Autodesk Fusion 360 part; units mm, degrees
(part 5 of 8)
  spline S1362 degree 3 poles (9.3996, -113.8343) (9.4042, -113.7081) (9.4002, -113.5528) (9.3979, -113.4927) knots 0 0 0 0 1 1 1 1
  spline S1363 degree 3 poles (9.3979, -113.4927) (9.3922, -113.4256) (9.399, -113.3996) (9.4154, -113.4303) knots 0 0 0 0 1 1 1 1
  spline S1364 degree 3 poles (9.4154, -113.4303) (9.4289, -113.4588) (9.4314, -113.4384) (9.4148, -113.3851) knots 0 0 0 0 1 1 1 1
  spline S1365 degree 3 poles (9.4148, -113.3851) (9.401, -113.334) (9.4015, -113.2762) (9.4145, -113.2595) knots 0 0 0 0 1 1 1 1
  spline S1366 degree 3 poles (9.4145, -113.2595) (9.4297, -113.24) (9.4323, -113.1794) (9.4222, -113.1178) knots 0 0 0 0 1 1 1 1
  spline S1367 degree 3 poles (9.4222, -113.1178) (9.4128, -113.0611) (9.4025, -112.9367) (9.4036, -112.8436) knots 0 0 0 0 1 1 1 1
  spline S1368 degree 3 poles (9.4036, -112.8436) (9.4042, -112.7455) (9.4014, -112.6001) (9.396, -112.5153) knots 0 0 0 0 1 1 1 1
  spline S1369 degree 3 poles (9.396, -112.5153) (9.3934, -112.4327) (9.3982, -112.3693) (9.4065, -112.3758) knots 0 0 0 0 1 1 1 1
  spline S1370 degree 3 poles (9.4065, -112.3758) (9.4176, -112.3845) (9.4227, -112.3437) (9.4154, -112.2842) knots 0 0 0 0 1 1 1 1
  spline S1371 degree 3 poles (9.4154, -112.2842) (9.4045, -112.1549) (9.4262, -112.1271) (9.5265, -112.1248) knots 0 0 0 0 1 1 1 1
  spline S1372 degree 3 poles (9.5265, -112.1248) (9.5992, -112.1234) (9.5964, -112.1213) (9.507, -112.1096) knots 0 0 0 0 1 1 1 1
  spline S1373 degree 3 poles (9.507, -112.1096) (9.4149, -112.0958) (9.4065, -112.0893) (9.3994, -111.9494) knots 0 0 0 0 1 1 1 1
  spline S1374 degree 3 poles (9.3994, -111.9494) (9.3946, -111.8696) (9.3998, -111.7885) (9.4106, -111.7746) knots 0 0 0 0 1 1 1 1
  spline S1375 degree 3 poles (9.4106, -111.7746) (9.4236, -111.7579) (9.4203, -111.7106) (9.405, -111.6672) knots 0 0 0 0 1 1 1 1
  spline S1376 degree 3 poles (9.405, -111.6672) (9.3896, -111.6239) (9.3885, -111.5738) (9.4037, -111.5543) knots 0 0 0 0 1 1 1 1
  spline S1377 degree 3 poles (9.4037, -111.5543) (9.4189, -111.5349) (9.4199, -111.4819) (9.4067, -111.4358) knots 0 0 0 0 1 1 1 1
  spline S1378 degree 3 poles (9.4067, -111.4358) (9.3935, -111.3897) (9.3902, -111.3423) (9.4011, -111.3284) knots 0 0 0 0 1 1 1 1
  spline S1379 degree 3 poles (9.4011, -111.3284) (9.4184, -111.3062) (9.4189, -111.2483) (9.4093, -111.0887) knots 0 0 0 0 1 1 1 1
  spline S1380 degree 3 poles (9.4093, -111.0887) (9.3971, -110.8866) (9.398, -110.5874) (9.4111, -110.5707) knots 0 0 0 0 1 1 1 1
  spline S1381 degree 3 poles (9.4111, -110.5707) (9.4176, -110.5624) (9.4208, -110.5067) (9.4185, -110.4467) knots 0 0 0 0 1 1 1 1
  spline S1382 degree 3 poles (9.4185, -110.4467) (9.406, -110.325) (9.4061, -110.2848) (9.3975, -109.9692) knots 0 0 0 0 1 1 1 1
  spline S1383 degree 3 poles (9.3975, -109.9692) (9.3922, -109.8442) (9.3981, -109.7279) (9.4068, -109.7167) knots 0 0 0 0 1 1 1 1
  spline S1384 degree 3 poles (9.4068, -109.7167) (9.4154, -109.7056) (9.4159, -109.6478) (9.4036, -109.589) knots 0 0 0 0 1 1 1 1
  spline S1385 degree 3 poles (9.4036, -109.589) (9.3942, -109.5323) (9.3967, -109.5119) (9.4102, -109.5404) knots 0 0 0 0 1 1 1 1
  spline S1386 degree 3 poles (9.4102, -109.5404) (9.426, -109.5661) (9.4282, -109.5231) (9.4207, -109.4411) knots 0 0 0 0 1 1 1 1
  spline S1387 degree 3 poles (9.4207, -109.4411) (9.3888, -109.161) (9.385, -109.1715) (9.5373, -109.1428) knots 0 0 0 0 1 1 1 1
  spline S1388 degree 3 poles (9.5373, -109.1428) (9.611, -109.1287) (9.6373, -109.1179) (9.5971, -109.1178) knots 0 0 0 0 1 1 1 1
  spline S1389 degree 3 poles (9.5971, -109.1178) (9.5569, -109.1178) (9.5136, -109.0929) (9.5056, -109.0688) knots 0 0 0 0 1 1 1 1
  spline S1390 degree 3 poles (9.5056, -109.0688) (9.4949, -109.0424) (9.4871, -109.0409) (9.483, -109.069) knots 0 0 0 0 1 1 1 1
  spline S1391 degree 3 poles (9.483, -109.069) (9.473, -109.1507) (9.4047, -109.1063) (9.3981, -109.0116) knots 0 0 0 0 1 1 1 1
  spline S1392 degree 3 poles (9.3981, -109.0116) (9.3942, -108.9593) (9.3998, -108.9234) (9.4109, -108.9321) knots 0 0 0 0 1 1 1 1
  spline S1393 degree 3 poles (9.4109, -108.9321) (9.4221, -108.9408) (9.4209, -108.8907) (9.4096, -108.8192) knots 0 0 0 0 1 1 1 1
  spline S1394 degree 3 poles (9.4096, -108.8192) (9.3983, -108.7477) (9.4, -108.6997) (9.4139, -108.7106) knots 0 0 0 0 1 1 1 1
  spline S1395 degree 3 poles (9.4139, -108.7106) (9.4278, -108.7214) (9.4235, -108.6868) (9.4097, -108.6357) knots 0 0 0 0 1 1 1 1
  spline S1396 degree 3 poles (9.4097, -108.6357) (9.3937, -108.5874) (9.392, -108.5323) (9.405, -108.5156) knots 0 0 0 0 1 1 1 1
  spline S1397 degree 3 poles (9.405, -108.5156) (9.4181, -108.4989) (9.4219, -108.4482) (9.4136, -108.4015) knots 0 0 0 0 1 1 1 1
  spline S1398 degree 3 poles (9.4136, -108.4015) (9.4054, -108.3547) (9.4002, -108.1895) (9.4033, -108.0308) knots 0 0 0 0 1 1 1 1
  spline S1399 degree 3 poles (9.4033, -108.0308) (9.4037, -107.8699) (9.3981, -107.7223) (9.3929, -107.7003) knots 0 0 0 0 1 1 1 1
  spline S1400 degree 3 poles (9.3929, -107.7003) (9.3843, -107.6712) (9.3908, -107.6629) (9.4103, -107.6781) knots 0 0 0 0 1 1 1 1
  spline S1401 degree 3 poles (9.4103, -107.6781) (9.4242, -107.6889) (9.4316, -107.6679) (9.4218, -107.6289) knots 0 0 0 0 1 1 1 1
  spline S1402 degree 3 poles (9.4218, -107.6289) (9.3982, -107.5388) (9.3926, -106.8584) (9.4148, -106.8758) knots 0 0 0 0 1 1 1 1
  spline S1403 degree 3 poles (9.4148, -106.8758) (9.4259, -106.8845) (9.4205, -106.8399) (9.4048, -106.774) knots 0 0 0 0 1 1 1 1
  spline S1404 degree 3 poles (9.4048, -106.774) (9.3898, -106.713) (9.3924, -106.6523) (9.4116, -106.645) knots 0 0 0 0 1 1 1 1
  spline S1405 degree 3 poles (9.4116, -106.645) (9.4336, -106.6397) (9.4339, -106.6221) (9.4145, -106.6069) knots 0 0 0 0 1 1 1 1
  spline S1406 degree 3 poles (9.4145, -106.6069) (9.3894, -106.5874) (9.396, -106.579) (9.4449, -106.568) knots 0 0 0 0 1 1 1 1
  spline S1407 degree 3 poles (9.4449, -106.568) (9.4987, -106.5564) (9.4953, -106.5492) (9.4338, -106.5191) knots 0 0 0 0 1 1 1 1
  spline S1408 degree 3 poles (9.4338, -106.5191) (9.3912, -106.4992) (9.3717, -106.484) (9.3888, -106.4794) knots 0 0 0 0 1 1 1 1
  spline S1409 degree 3 poles (9.3888, -106.4794) (9.4036, -106.4776) (9.4125, -106.386) (9.4013, -106.2743) knots 0 0 0 0 1 1 1 1
  spline S1410 degree 3 poles (9.4013, -106.2743) (9.3928, -106.1647) (9.3977, -106.0611) (9.4151, -106.0388) knots 0 0 0 0 1 1 1 1
  spline S1411 degree 3 poles (9.4151, -106.0388) (9.4303, -106.0194) (9.4322, -105.994) (9.4183, -105.9832) knots 0 0 0 0 1 1 1 1
  spline S1412 degree 3 poles (9.4183, -105.9832) (9.3877, -105.9593) (9.3954, -105.2848) (9.4254, -105.2635) knots 0 0 0 0 1 1 1 1
  spline S1413 degree 3 poles (9.4254, -105.2635) (9.4397, -105.2567) (9.44, -105.2391) (9.4261, -105.2282) knots 0 0 0 0 1 1 1 1
  spline S1414 degree 3 poles (9.4261, -105.2282) (9.3733, -105.187) (9.3985, -104.6963) (9.4496, -104.6825) knots 0 0 0 0 1 1 1 1
  spline S1415 degree 3 poles (9.4496, -104.6825) (9.4815, -104.676) (9.5088, -104.6526) (9.5212, -104.631) knots 0 0 0 0 1 1 1 1
  spline S1416 degree 3 poles (11.4691, -103.9771) (11.4765, -103.9963) (11.5151, -104.0041) (11.5542, -103.9943) knots 0 0 0 0 1 1 1 1
  spline S1417 degree 3 poles (11.5542, -103.9943) (11.6179, -103.9814) (11.6223, -103.9759) (11.5687, -103.9699) knots 0 0 0 0 1 1 1 1
  spline S1418 degree 3 poles (11.5687, -103.9699) (11.5152, -103.9639) (11.5174, -103.9611) (11.5833, -103.9455) knots 0 0 0 0 1 1 1 1
  spline S1419 degree 3 poles (11.5833, -103.9455) (11.6713, -103.9246) (11.7334, -103.9597) (11.6637, -103.9859) knots 0 0 0 0 1 1 1 1
  spline S1420 degree 3 poles (11.6637, -103.9859) (11.6281, -104.0028) (11.6336, -104.0072) (11.6832, -104.0011) knots 0 0 0 0 1 1 1 1
  spline S1421 degree 3 poles (11.6832, -104.0011) (11.7206, -103.999) (11.7612, -103.9814) (11.7742, -103.9648) knots 0 0 0 0 1 1 1 1
  spline S1422 degree 3 poles (11.7742, -103.9648) (11.7872, -103.9481) (11.8191, -103.9417) (11.8479, -103.9507) knots 0 0 0 0 1 1 1 1
  spline S1423 degree 3 poles (11.8479, -103.9507) (11.8794, -103.9619) (11.8785, -103.9746) (11.8422, -103.9866) knots 0 0 0 0 1 1 1 1
  spline S1424 degree 3 poles (11.8422, -103.9866) (11.7995, -104.0069) (11.8023, -104.0091) (11.8672, -104.0061) knots 0 0 0 0 1 1 1 1
  spline S1425 degree 3 poles (11.8672, -104.0061) (11.9124, -104.0056) (11.9437, -103.9942) (11.9419, -103.9794) knots 0 0 0 0 1 1 1 1
  spline S1426 degree 3 poles (11.9419, -103.9794) (11.9404, -103.9469) (12.0531, -103.923) (12.0864, -103.9491) knots 0 0 0 0 1 1 1 1
  spline S1427 degree 3 poles (12.0864, -103.9491) (12.1003, -103.9599) (12.0944, -103.9732) (12.0731, -103.9834) knots 0 0 0 0 1 1 1 1
  spline S1428 degree 3 poles (12.0731, -103.9834) (12.0105, -104.0061) (12.0519, -104.0161) (12.1327, -103.9987) knots 0 0 0 0 1 1 1 1
  spline S1429 degree 3 poles (12.1327, -103.9987) (12.1987, -103.983) (12.2008, -103.9802) (12.1473, -103.9742) knots 0 0 0 0 1 1 1 1
  spline S1430 degree 3 poles (12.1473, -103.9742) (12.0938, -103.9683) (12.096, -103.9655) (12.1619, -103.9498) knots 0 0 0 0 1 1 1 1
  spline S1431 degree 3 poles (12.1619, -103.9498) (12.2399, -103.9302) (12.3141, -103.9613) (12.2494, -103.9868) knots 0 0 0 0 1 1 1 1
  spline S1432 degree 3 poles (12.2494, -103.9868) (12.1797, -104.013) (12.2283, -104.0196) (12.3338, -103.9991) knots 0 0 0 0 1 1 1 1
  spline S1433 degree 3 poles (12.3338, -103.9991) (12.4344, -103.9792) (12.4366, -103.9764) (12.3484, -103.9747) knots 0 0 0 0 1 1 1 1
  spline S1434 degree 3 poles (12.3484, -103.9747) (12.2603, -103.9729) (12.2624, -103.9702) (12.363, -103.9503) knots 0 0 0 0 1 1 1 1
  spline S1435 degree 3 poles (12.363, -103.9503) (12.4686, -103.9298) (12.5471, -103.9553) (12.4682, -103.9876) knots 0 0 0 0 1 1 1 1
  spline S1436 degree 3 poles (12.4682, -103.9876) (12.4319, -103.9996) (12.4403, -104.0061) (12.4932, -104.0072) knots 0 0 0 0 1 1 1 1
  spline S1437 degree 3 poles (12.4932, -104.0072) (12.5356, -104.0045) (12.5761, -103.9869) (12.5842, -103.9709) knots 0 0 0 0 1 1 1 1
  spline S1438 degree 3 poles (12.5842, -103.9709) (12.5945, -103.952) (12.6236, -103.9434) (12.6523, -103.9525) knots 0 0 0 0 1 1 1 1
  spline S1439 degree 3 poles (12.6523, -103.9525) (12.6839, -103.9637) (12.6829, -103.9763) (12.6495, -103.9905) knots 0 0 0 0 1 1 1 1
  spline S1440 degree 3 poles (12.6495, -103.9905) (12.6182, -104.0019) (12.6392, -104.0094) (12.6965, -104.0048) knots 0 0 0 0 1 1 1 1
  spline S1441 degree 3 poles (12.6965, -104.0048) (12.7515, -104.0031) (12.802, -103.9843) (12.8144, -103.9627) knots 0 0 0 0 1 1 1 1
  spline S1442 degree 3 poles (12.8144, -103.9627) (12.8247, -103.9439) (12.8528, -103.9479) (12.8779, -103.9675) knots 0 0 0 0 1 1 1 1
  spline S1443 degree 3 poles (12.8779, -103.9675) (12.9035, -103.992) (12.9267, -103.9967) (12.927, -103.979) knots 0 0 0 0 1 1 1 1
  spline S1444 degree 3 poles (12.927, -103.979) (12.9336, -103.9305) (13.0725, -103.936) (13.0737, -103.9862) knots 0 0 0 0 1 1 1 1
  spline S1445 degree 3 poles (13.0737, -103.9862) (13.0871, -104.3414) (13.0769, -104.5035) (13.0385, -104.5183) knots 0 0 0 0 1 1 1 1
  spline S1446 degree 3 poles (13.0385, -104.5183) (13.0121, -104.529) (13.0106, -104.5368) (13.0338, -104.5415) knots 0 0 0 0 1 1 1 1
  spline S1447 degree 3 poles (13.0338, -104.5415) (13.0669, -104.5449) (13.0985, -106.3783) (13.0691, -106.5075) knots 0 0 0 0 1 1 1 1
  spline S1448 degree 3 poles (13.0691, -106.5075) (13.0654, -106.518) (12.8203, -106.528) (12.526, -106.5264) knots 0 0 0 0 1 1 1 1
  spline S1449 degree 3 poles (12.526, -106.5264) (12.2318, -106.5249) (11.9861, -106.5299) (11.9818, -106.5355) knots 0 0 0 0 1 1 1 1
  spline S1450 degree 3 poles (11.9818, -106.5355) (11.9753, -106.5438) (12.0365, -106.5514) (12.117, -106.5515) knots 0 0 0 0 1 1 1 1
  spline S1451 degree 3 poles (12.117, -106.5515) (12.2023, -106.5511) (12.2735, -106.5575) (12.2846, -106.5661) knots 0 0 0 0 1 1 1 1
  spline S1452 degree 3 poles (12.2846, -106.5661) (12.293, -106.5727) (12.3018, -106.9109) (12.3059, -107.3125) knots 0 0 0 0 1 1 1 1
  spline S1453 degree 3 poles (12.3059, -107.3125) (12.3107, -107.7819) (12.333, -108.0857) (12.3678, -108.1443) knots 0 0 0 0 1 1 1 1
  spline S1454 degree 3 poles (12.3678, -108.1443) (12.3965, -108.1936) (12.5461, -108.4089) (12.7028, -108.6209) knots 0 0 0 0 1 1 1 1
  spline S1455 degree 3 poles (12.7028, -108.6209) (12.8546, -108.8335) (12.9902, -109.038) (12.9951, -109.0776) knots 0 0 0 0 1 1 1 1
  spline S1456 degree 3 poles (12.9951, -109.0776) (13.007, -109.1541) (12.959, -109.1926) (12.546, -109.4519) knots 0 0 0 0 1 1 1 1
  spline S1457 degree 3 poles (12.546, -109.4519) (12.3895, -109.5491) (12.3055, -109.6222) (12.2961, -109.6686) knots 0 0 0 0 1 1 1 1
  spline S1458 degree 3 poles (12.2961, -109.6686) (12.2855, -109.7051) (12.3057, -109.9715) (12.3403, -110.2538) knots 0 0 0 0 1 1 1 1
  line L112 (12.3403, -110.2538) -> (12.3986, -110.7694)
  line L113 (12.3986, -110.7694) -> (12.6643, -111.2143)
  line L114 (12.6643, -111.2143) -> (12.9273, -111.657)
  line L115 (12.9273, -111.657) -> (12.9828, -112.1704)
  spline S1459 degree 3 poles (12.9828, -112.1704) (13.0278, -112.5369) (13.028, -112.7027) (12.9911, -112.75) knots 0 0 0 0 1 1 1 1
  spline S1460 degree 3 poles (12.9911, -112.75) (12.9607, -112.7889) (12.7218, -112.9514) (12.4554, -113.1148) knots 0 0 0 0 1 1 1 1
  spline S1461 degree 3 poles (12.4554, -113.1148) (12.126, -113.3186) (11.9599, -113.4395) (11.9205, -113.5072) knots 0 0 0 0 1 1 1 1
  spline S1462 degree 3 poles (11.9205, -113.5072) (11.8605, -113.6126) (11.7411, -114.2983) (11.7541, -114.4651) knots 0 0 0 0 1 1 1 1
  spline S1463 degree 3 poles (11.7541, -114.4651) (11.7564, -114.5251) (11.7792, -114.5877) (11.8014, -114.605) knots 0 0 0 0 1 1 1 1
  spline S1464 degree 3 poles (11.8014, -114.605) (11.8264, -114.6246) (11.8217, -114.6478) (11.7889, -114.6669) knots 0 0 0 0 1 1 1 1
  spline S1465 degree 3 poles (11.7889, -114.6669) (11.7468, -114.6922) (11.7502, -114.6993) (11.7926, -114.6966) knots 0 0 0 0 1 1 1 1
  spline S1466 degree 3 poles (11.7926, -114.6966) (11.8752, -114.694) (12.6789, -116.1636) (12.6604, -116.279) knots 0 0 0 0 1 1 1 1
  spline S1467 degree 3 poles (12.6604, -116.279) (12.6538, -116.3275) (12.4805, -116.6353) (12.2799, -116.9666) knots 0 0 0 0 1 1 1 1
  spline S1468 degree 3 poles (12.2799, -116.9666) (12.0641, -117.3173) (11.9087, -117.6078) (11.9049, -117.6585) knots 0 0 0 0 1 1 1 1
  spline S1469 degree 3 poles (11.9049, -117.6585) (11.8973, -117.7197) (12.0151, -117.9415) (12.2824, -118.3787) knots 0 0 0 0 1 1 1 1
  spline S1470 degree 3 poles (12.2824, -118.3787) (12.735, -119.1173) (12.7463, -119.0053) (12.1724, -119.4478) knots 0 0 0 0 1 1 1 1
  spline S1471 degree 3 poles (12.1724, -119.4478) (11.789, -119.7437) (11.7111, -119.8261) (11.6907, -119.9668) knots 0 0 0 0 1 1 1 1
  spline S1472 degree 3 poles (11.6907, -119.9668) (11.6626, -120.106) (11.7858, -120.7619) (11.8564, -120.8663) knots 0 0 0 0 1 1 1 1
  spline S1473 degree 3 poles (11.8564, -120.8663) (11.9742, -121.0479) (12.5647, -122.1315) (12.5714, -122.186) knots 0 0 0 0 1 1 1 1
  spline S1474 degree 3 poles (12.5714, -122.186) (12.5756, -122.2206) (12.4475, -122.3846) (12.1544, -122.7197) knots 0 0 0 0 1 1 1 1
  spline S1475 degree 3 poles (12.1544, -122.7197) (11.8237, -123.0971) (11.7086, -123.2444) (11.643, -123.3857) knots 0 0 0 0 1 1 1 1
  spline S1476 degree 3 poles (11.643, -123.3857) (11.5694, -123.543) (11.4368, -123.7528) (11.4341, -123.7104) knots 0 0 0 0 1 1 1 1
  spline S1477 degree 3 poles (11.4341, -123.7104) (11.4295, -122.5473) (11.4436, -122.1912) (11.4873, -122.1582) knots 0 0 0 0 1 1 1 1
  spline S1478 degree 3 poles (11.4873, -122.1582) (11.5245, -122.1336) (11.5239, -122.1286) (11.4898, -122.1378) knots 0 0 0 0 1 1 1 1
  spline S1479 degree 3 poles (11.4898, -122.1378) (11.4536, -122.1498) (11.4365, -121.7649) (11.4348, -120.8502) knots 0 0 0 0 1 1 1 1
  spline S1480 degree 3 poles (11.4348, -120.8502) (11.4348, -119.8475) (11.4478, -119.5443) (11.4936, -119.5487) knots 0 0 0 0 1 1 1 1
  spline S1481 degree 3 poles (11.4936, -119.5487) (11.5388, -119.5482) (11.5382, -119.5432) (11.4912, -119.5289) knots 0 0 0 0 1 1 1 1
  spline S1482 degree 3 poles (11.4912, -119.5289) (11.4513, -119.5112) (11.4341, -119.453) (11.4328, -119.34) knots 0 0 0 0 1 1 1 1
  spline S1483 degree 3 poles (11.4328, -119.34) (11.4345, -119.2518) (11.4338, -118.7543) (11.4312, -118.2419) knots 0 0 0 0 1 1 1 1
  spline S1484 degree 3 poles (11.4312, -118.2419) (11.4303, -117.4981) (11.4447, -117.3079) (11.4926, -117.3095) knots 0 0 0 0 1 1 1 1
  spline S1485 degree 3 poles (11.4926, -117.3095) (11.5406, -117.3112) (11.5427, -117.3084) (11.4951, -117.2891) knots 0 0 0 0 1 1 1 1
  spline S1486 degree 3 poles (11.4951, -117.2891) (11.4509, -117.2769) (11.4364, -116.9746) (11.4365, -116.0749) knots 0 0 0 0 1 1 1 1
  spline S1487 degree 3 poles (11.4365, -116.0749) (11.4361, -115.4164) (11.4358, -114.0015) (11.435, -112.931) knots 0 0 0 0 1 1 1 1
  spline S1488 degree 3 poles (11.435, -112.931) (11.4349, -111.8654) (11.4321, -110.5739) (11.4351, -110.0659) knots 0 0 0 0 1 1 1 1
  spline S1489 degree 3 poles (11.4351, -110.0659) (11.4299, -109.3276) (11.4448, -109.1423) (11.4937, -109.1313) knots 0 0 0 0 1 1 1 1
  spline S1490 degree 3 poles (11.4937, -109.1313) (11.5448, -109.1174) (11.5464, -109.1097) (11.4994, -109.0954) knots 0 0 0 0 1 1 1 1
  spline S1491 degree 3 poles (11.4994, -109.0954) (11.4552, -109.0832) (11.438, -109.025) (11.4367, -108.9121) knots 0 0 0 0 1 1 1 1
  spline S1492 degree 3 poles (11.4367, -108.9121) (11.4356, -108.8217) (11.4349, -108.1809) (11.4358, -107.4922) knots 0 0 0 0 1 1 1 1
  spline S1493 degree 3 poles (11.4358, -107.4922) (11.4339, -106.8013) (11.4353, -105.728) (11.4342, -105.1048) knots 0 0 0 0 1 1 1 1
  spline S1494 degree 3 poles (11.4342, -105.1048) (11.4352, -104.4789) (11.4397, -103.9631) (11.4441, -103.9576) knots 0 0 0 0 1 1 1 1
  spline S1495 degree 3 poles (11.4441, -103.9576) (11.4506, -103.9492) (11.4617, -103.9579) (11.4691, -103.9771) knots 0 0 0 0 1 1 1 1
  spline S1496 degree 3 poles (10.2121, -106.2049) (10.2283, -106.2758) (10.2333, -106.2752) (10.2319, -106.2024) knots 0 0 0 0 1 1 1 1
  spline S1497 degree 3 poles (10.2319, -106.2024) (10.232, -106.1622) (10.2271, -106.1226) (10.2215, -106.1183) knots 0 0 0 0 1 1 1 1
  spline S1498 degree 3 poles (10.2215, -106.1183) (10.1993, -106.1009) (10.1958, -106.134) (10.2121, -106.2049) knots 0 0 0 0 1 1 1 1
  spline S1499 degree 3 poles (9.9148, -109.1467) (9.9204, -109.151) (9.96, -109.1462) (10.0012, -109.1336) knots 0 0 0 0 1 1 1 1
  spline S1500 degree 3 poles (10.0012, -109.1336) (10.0699, -109.1201) (10.0693, -109.1152) (9.9966, -109.1165) knots 0 0 0 0 1 1 1 1
  spline S1501 degree 3 poles (9.9966, -109.1165) (9.9238, -109.1179) (9.8926, -109.1293) (9.9148, -109.1467) knots 0 0 0 0 1 1 1 1
  spline S1502 degree 3 poles (9.4857, -110.1142) (9.502, -110.1851) (9.5069, -110.1845) (9.5055, -110.1118) knots 0 0 0 0 1 1 1 1
  spline S1503 degree 3 poles (9.5055, -110.1118) (9.5056, -110.0715) (9.5007, -110.0319) (9.4952, -110.0276) knots 0 0 0 0 1 1 1 1
  spline S1504 degree 3 poles (9.4952, -110.0276) (9.4729, -110.0102) (9.4695, -110.0433) (9.4857, -110.1142) knots 0 0 0 0 1 1 1 1
  spline S1505 degree 3 poles (10.2155, -110.3262) (10.2317, -110.3971) (10.2366, -110.3965) (10.2353, -110.3238) knots 0 0 0 0 1 1 1 1
  spline S1506 degree 3 poles (10.2353, -110.3238) (10.2353, -110.2835) (10.2305, -110.2439) (10.2249, -110.2396) knots 0 0 0 0 1 1 1 1
  spline S1507 degree 3 poles (10.2249, -110.2396) (10.2027, -110.2222) (10.1992, -110.2553) (10.2155, -110.3262) knots 0 0 0 0 1 1 1 1
  spline S1508 degree 3 poles (9.7288, -112.1352) (9.7344, -112.1395) (9.774, -112.1346) (9.8152, -112.122) knots 0 0 0 0 1 1 1 1
  spline S1509 degree 3 poles (9.8152, -112.122) (9.8839, -112.1086) (9.8833, -112.1036) (9.8106, -112.105) knots 0 0 0 0 1 1 1 1
  spline S1510 degree 3 poles (9.8106, -112.105) (9.7379, -112.1064) (9.7066, -112.1178) (9.7288, -112.1352) knots 0 0 0 0 1 1 1 1
  spline S1511 degree 3 poles (9.4874, -113.6074) (9.5036, -113.6783) (9.5086, -113.6777) (9.5072, -113.605) knots 0 0 0 0 1 1 1 1
  spline S1512 degree 3 poles (9.5072, -113.605) (9.5058, -113.5323) (9.4944, -113.501) (9.477, -113.5232) knots 0 0 0 0 1 1 1 1
  spline S1513 degree 3 poles (9.477, -113.5232) (9.4727, -113.5288) (9.4776, -113.5684) (9.4874, -113.6074) knots 0 0 0 0 1 1 1 1
  spline S1514 degree 3 poles (9.4865, -114.0096) (9.5027, -114.0805) (9.5077, -114.0799) (9.5063, -114.0072) knots 0 0 0 0 1 1 1 1
  spline S1515 degree 3 poles (9.5063, -114.0072) (9.5064, -113.967) (9.5015, -113.9274) (9.496, -113.923) knots 0 0 0 0 1 1 1 1
  spline S1516 degree 3 poles (9.496, -113.923) (9.4737, -113.9057) (9.4703, -113.9387) (9.4865, -114.0096) knots 0 0 0 0 1 1 1 1
  spline S1517 degree 3 poles (9.4856, -114.4119) (9.5019, -114.4828) (9.5068, -114.4821) (9.5054, -114.4094) knots 0 0 0 0 1 1 1 1
  spline S1518 degree 3 poles (9.5054, -114.4094) (9.504, -114.3367) (9.4927, -114.3054) (9.4753, -114.3277) knots 0 0 0 0 1 1 1 1
  spline S1519 degree 3 poles (9.4753, -114.3277) (9.4709, -114.3332) (9.4758, -114.3729) (9.4856, -114.4119) knots 0 0 0 0 1 1 1 1
  spline S1520 degree 3 poles (9.9086, -114.8274) (9.9142, -114.8317) (9.9538, -114.8269) (9.995, -114.8143) knots 0 0 0 0 1 1 1 1
  spline S1521 degree 3 poles (9.995, -114.8143) (10.0637, -114.8008) (10.0631, -114.7959) (9.9903, -114.7973) knots 0 0 0 0 1 1 1 1
  spline S1522 degree 3 poles (9.9903, -114.7973) (9.9176, -114.7986) (9.8864, -114.81) (9.9086, -114.8274) knots 0 0 0 0 1 1 1 1
  spline S1523 degree 3 poles (9.4882, -116.0703) (9.5044, -116.1412) (9.5094, -116.1406) (9.508, -116.0679) knots 0 0 0 0 1 1 1 1
  spline S1524 degree 3 poles (9.508, -116.0679) (9.5066, -115.9952) (9.4952, -115.9639) (9.4779, -115.9861) knots 0 0 0 0 1 1 1 1
  spline S1525 degree 3 poles (9.4779, -115.9861) (9.4735, -115.9917) (9.4784, -116.0313) (9.4882, -116.0703) knots 0 0 0 0 1 1 1 1
  spline S1526 degree 3 poles (9.489, -117.1006) (9.5053, -117.1715) (9.5102, -117.1709) (9.5088, -117.0982) knots 0 0 0 0 1 1 1 1
  spline S1527 degree 3 poles (9.5088, -117.0982) (9.5089, -117.058) (9.5041, -117.0184) (9.4985, -117.014) knots 0 0 0 0 1 1 1 1
  spline S1528 degree 3 poles (9.4985, -117.014) (9.4763, -116.9966) (9.4728, -117.0297) (9.489, -117.1006) knots 0 0 0 0 1 1 1 1
  spline S1529 degree 3 poles (10.2118, -116.2328) (10.2281, -116.3037) (10.233, -116.303) (10.2317, -116.2303) knots 0 0 0 0 1 1 1 1
  spline S1530 degree 3 poles (10.2317, -116.2303) (10.2303, -116.1576) (10.2189, -116.1263) (10.2015, -116.1486) knots 0 0 0 0 1 1 1 1
  spline S1531 degree 3 poles (10.2015, -116.1486) (10.1972, -116.1541) (10.202, -116.1938) (10.2118, -116.2328) knots 0 0 0 0 1 1 1 1
  spline S1532 degree 3 poles (9.4847, -117.6792) (9.5009, -117.7501) (9.5059, -117.7495) (9.5045, -117.6768) knots 0 0 0 0 1 1 1 1
  spline S1533 degree 3 poles (9.5045, -117.6768) (9.5046, -117.6366) (9.4997, -117.5969) (9.4941, -117.5926) knots 0 0 0 0 1 1 1 1
  spline S1534 degree 3 poles (9.4941, -117.5926) (9.4719, -117.5752) (9.4684, -117.6083) (9.4847, -117.6792) knots 0 0 0 0 1 1 1 1
  spline S1535 degree 3 poles (9.7669, -117.358) (9.7725, -117.3624) (9.8121, -117.3575) (9.8533, -117.3449) knots 0 0 0 0 1 1 1 1
  spline S1536 degree 3 poles (9.8533, -117.3449) (9.922, -117.3315) (9.9214, -117.3265) (9.8487, -117.3279) knots 0 0 0 0 1 1 1 1
  spline S1537 degree 3 poles (9.8487, -117.3279) (9.776, -117.3293) (9.7447, -117.3407) (9.7669, -117.358) knots 0 0 0 0 1 1 1 1
  spline S1538 degree 3 poles (9.9433, -117.3615) (9.9489, -117.3659) (9.9885, -117.361) (10.0296, -117.3484) knots 0 0 0 0 1 1 1 1
  spline S1539 degree 3 poles (10.0296, -117.3484) (10.0984, -117.3349) (10.0978, -117.33) (10.025, -117.3314) knots 0 0 0 0 1 1 1 1
  spline S1540 degree 3 poles (10.025, -117.3314) (9.9523, -117.3328) (9.9211, -117.3441) (9.9433, -117.3615) knots 0 0 0 0 1 1 1 1
  spline S1541 degree 3 poles (9.4864, -118.3073) (9.5026, -118.3782) (9.5076, -118.3776) (9.5062, -118.3049) knots 0 0 0 0 1 1 1 1
  spline S1542 degree 3 poles (9.5062, -118.3049) (9.5063, -118.2647) (9.5014, -118.225) (9.4959, -118.2207) knots 0 0 0 0 1 1 1 1
  spline S1543 degree 3 poles (9.4959, -118.2207) (9.4736, -118.2033) (9.4702, -118.2364) (9.4864, -118.3073) knots 0 0 0 0 1 1 1 1
  spline S1544 degree 3 poles (9.793, -119.6168) (9.7985, -119.6211) (9.8381, -119.6162) (9.8793, -119.6037) knots 0 0 0 0 1 1 1 1
  spline S1545 degree 3 poles (9.8793, -119.6037) (9.948, -119.5902) (9.9474, -119.5852) (9.8747, -119.5866) knots 0 0 0 0 1 1 1 1
  spline S1546 degree 3 poles (9.8747, -119.5866) (9.802, -119.588) (9.7707, -119.5994) (9.793, -119.6168) knots 0 0 0 0 1 1 1 1
  spline S1547 degree 3 poles (10.0188, -119.6142) (10.0244, -119.6185) (10.064, -119.6136) (10.1052, -119.6011) knots 0 0 0 0 1 1 1 1
  spline S1548 degree 3 poles (10.1052, -119.6011) (10.1739, -119.5876) (10.1733, -119.5826) (10.1006, -119.584) knots 0 0 0 0 1 1 1 1
  spline S1549 degree 3 poles (10.1006, -119.584) (10.0279, -119.5854) (9.9966, -119.5968) (10.0188, -119.6142) knots 0 0 0 0 1 1 1 1
  spline S1550 degree 3 poles (10.2058, -119.5812) (10.2029, -119.6192) (10.2119, -119.6307) (10.2271, -119.6112) knots 0 0 0 0 1 1 1 1
  spline S1551 degree 3 poles (10.2271, -119.6112) (10.2401, -119.5945) (10.2457, -119.5587) (10.2384, -119.5395) knots 0 0 0 0 1 1 1 1
  spline S1552 degree 3 poles (10.2384, -119.5395) (10.2224, -119.4912) (10.2137, -119.5023) (10.2058, -119.5812) knots 0 0 0 0 1 1 1 1
  spline S1553 degree 3 poles (10.2152, -120.3541) (10.2315, -120.425) (10.2364, -120.4244) (10.235, -120.3516) knots 0 0 0 0 1 1 1 1
  spline S1554 degree 3 poles (10.235, -120.3516) (10.2351, -120.3114) (10.2303, -120.2718) (10.2247, -120.2675) knots 0 0 0 0 1 1 1 1
  spline S1555 degree 3 poles (10.2247, -120.2675) (10.2025, -120.2501) (10.199, -120.2832) (10.2152, -120.3541) knots 0 0 0 0 1 1 1 1
  spline S1556 degree 3 poles (9.4855, -121.5746) (9.5017, -121.6455) (9.5067, -121.6449) (9.5053, -121.5722) knots 0 0 0 0 1 1 1 1
  spline S1557 degree 3 poles (9.5053, -121.5722) (9.5054, -121.532) (9.5005, -121.4924) (9.4949, -121.488) knots 0 0 0 0 1 1 1 1
  spline S1558 degree 3 poles (9.4949, -121.488) (9.4727, -121.4707) (9.4692, -121.5038) (9.4855, -121.5746) knots 0 0 0 0 1 1 1 1
  spline S1559 degree 3 poles (9.4699, -122.1848) (9.4639, -122.2383) (9.4871, -122.243) (9.6053, -122.2234) knots 0 0 0 0 1 1 1 1
  spline S1560 degree 3 poles (9.6053, -122.2234) (9.6846, -122.2137) (9.701, -122.2041) (9.6459, -122.2059) knots 0 0 0 0 1 1 1 1
  spline S1561 degree 3 poles (9.6459, -122.2059) (9.5908, -122.2076) (9.5305, -122.1874) (9.512, -122.1595) knots 0 0 0 0 1 1 1 1
  spline S1562 degree 3 poles (9.512, -122.1595) (9.4772, -122.1009) (9.4772, -122.1009) (9.4699, -122.1848) knots 0 0 0 0 1 1 1 1
  spline S1563 degree 3 poles (9.4898, -122.4286) (9.506, -122.4995) (9.511, -122.4989) (9.5096, -122.4262) knots 0 0 0 0 1 1 1 1
  spline S1564 degree 3 poles (9.5096, -122.4262) (9.5097, -122.386) (9.5048, -122.3464) (9.4993, -122.342) knots 0 0 0 0 1 1 1 1
  spline S1565 degree 3 poles (9.4993, -122.342) (9.477, -122.3246) (9.4735, -122.3577) (9.4898, -122.4286) knots 0 0 0 0 1 1 1 1
  spline S1566 degree 3 poles (9.7625, -122.2343) (9.768, -122.2386) (9.8077, -122.2338) (9.8488, -122.2212) knots 0 0 0 0 1 1 1 1
  spline S1567 degree 3 poles (9.8488, -122.2212) (9.9176, -122.2077) (9.917, -122.2028) (9.8442, -122.2041) knots 0 0 0 0 1 1 1 1
  spline S1568 degree 3 poles (9.8442, -122.2041) (9.7715, -122.2055) (9.7402, -122.2169) (9.7625, -122.2343) knots 0 0 0 0 1 1 1 1
  spline S1569 degree 3 poles (10.2117, -121.963) (10.228, -122.0339) (10.2329, -122.0333) (10.2315, -121.9606) knots 0 0 0 0 1 1 1 1
  spline S1570 degree 3 poles (10.2315, -121.9606) (10.2316, -121.9203) (10.2268, -121.8807) (10.2212, -121.8764) knots 0 0 0 0 1 1 1 1
  spline S1571 degree 3 poles (10.2212, -121.8764) (10.199, -121.859) (10.1955, -121.8921) (10.2117, -121.963) knots 0 0 0 0 1 1 1 1
  spline S1572 degree 3 poles (9.9884, -122.2317) (9.9939, -122.236) (10.0335, -122.2312) (10.0747, -122.2186) knots 0 0 0 0 1 1 1 1
  spline S1573 degree 3 poles (10.0747, -122.2186) (10.1434, -122.2051) (10.1428, -122.2002) (10.0701, -122.2015) knots 0 0 0 0 1 1 1 1
  spline S1574 degree 3 poles (10.0701, -122.2015) (9.9974, -122.2029) (9.9661, -122.2143) (9.9884, -122.2317) knots 0 0 0 0 1 1 1 1
  spline S1575 degree 3 poles (11.4718, -106.5579) (11.4857, -106.5687) (11.5105, -106.5657) (11.5235, -106.549) knots 0 0 0 0 1 1 1 1
  spline S1576 degree 3 poles (11.5235, -106.549) (11.5344, -106.5351) (11.5248, -106.5187) (11.5044, -106.5162) knots 0 0 0 0 1 1 1 1
  spline S1577 degree 3 poles (11.5044, -106.5162) (11.4812, -106.5115) (11.4592, -106.5167) (11.4527, -106.525) knots 0 0 0 0 1 1 1 1
  spline S1578 degree 3 poles (11.4527, -106.525) (11.4484, -106.5306) (11.4551, -106.5448) (11.4718, -106.5579) knots 0 0 0 0 1 1 1 1
  spline S1579 degree 3 poles (11.4752, -112.1117) (11.4891, -112.1226) (11.5138, -112.1196) (11.5269, -112.1029) knots 0 0 0 0 1 1 1 1
  spline S1580 degree 3 poles (11.5269, -112.1029) (11.5377, -112.089) (11.5282, -112.0726) (11.5078, -112.07) knots 0 0 0 0 1 1 1 1
  spline S1581 degree 3 poles (11.5078, -112.07) (11.4846, -112.0654) (11.4626, -112.0706) (11.4561, -112.0789) knots 0 0 0 0 1 1 1 1
  spline S1582 degree 3 poles (11.4561, -112.0789) (11.4517, -112.0845) (11.4585, -112.0987) (11.4752, -112.1117) knots 0 0 0 0 1 1 1 1
  spline S1583 degree 3 poles (11.4814, -114.8027) (11.4953, -114.8135) (11.5117, -114.804) (11.5142, -114.7836) knots 0 0 0 0 1 1 1 1
  spline S1584 degree 3 poles (11.5142, -114.7836) (11.5189, -114.7604) (11.5137, -114.7384) (11.5054, -114.7319) knots 0 0 0 0 1 1 1 1
  spline S1585 degree 3 poles (11.5054, -114.7319) (11.4998, -114.7275) (11.4855, -114.7343) (11.4725, -114.751) knots 0 0 0 0 1 1 1 1
  spline S1586 degree 3 poles (11.4725, -114.751) (11.4617, -114.7649) (11.4647, -114.7896) (11.4814, -114.8027) knots 0 0 0 0 1 1 1 1
  line L116 (11.4894, -114.9701) -> (11.512, -115.0729)
  line L117 (11.512, -115.0729) -> (11.5092, -114.9676)
  spline S1587 degree 3 poles (11.5092, -114.9676) (11.5047, -114.8702) (11.4955, -114.8361) (11.4782, -114.8584) knots 0 0 0 0 1 1 1 1
  spline S1588 degree 3 poles (11.4782, -114.8584) (11.4738, -114.8639) (11.4799, -114.9134) (11.4894, -114.9701) knots 0 0 0 0 1 1 1 1
  spline S1589 degree 3 poles (11.4889, -115.1712) (11.5052, -115.2421) (11.5101, -115.2415) (11.5087, -115.1688) knots 0 0 0 0 1 1 1 1
  spline S1590 degree 3 poles (11.5087, -115.1688) (11.5073, -115.096) (11.496, -115.0648) (11.4786, -115.087) knots 0 0 0 0 1 1 1 1
  spline S1591 degree 3 poles (11.4786, -115.087) (11.4742, -115.0926) (11.4791, -115.1322) (11.4889, -115.1712) knots 0 0 0 0 1 1 1 1
  spline S1592 degree 3 poles (10.3862, -94.1953) (10.432, -94.1997) (10.4886, -94.1903) (10.5165, -94.1718) knots 0 0 0 0 1 1 1 1
  spline S1593 degree 3 poles (10.5165, -94.1718) (10.545, -94.1582) (10.5113, -94.1498) (10.4441, -94.1555) knots 0 0 0 0 1 1 1 1
  spline S1594 degree 3 poles (10.4441, -94.1555) (10.295, -94.1688) (10.2742, -94.1839) (10.3862, -94.1953) knots 0 0 0 0 1 1 1 1
  spline S1595 degree 3 poles (10.5328, -93.9159) (10.5384, -93.9203) (10.578, -93.9154) (10.6192, -93.9028) knots 0 0 0 0 1 1 1 1
  spline S1596 degree 3 poles (10.6192, -93.9028) (10.6879, -93.8893) (10.6873, -93.8844) (10.6146, -93.8858) knots 0 0 0 0 1 1 1 1
  spline S1597 degree 3 poles (10.6146, -93.8858) (10.5419, -93.8872) (10.5106, -93.8985) (10.5328, -93.9159) knots 0 0 0 0 1 1 1 1
  spline S1598 degree 3 poles (14.1501, -89.3777) (14.2024, -89.3738) (14.2491, -89.3655) (14.2557, -89.3572) knots 0 0 0 0 1 1 1 1
  spline S1599 degree 3 poles (14.2557, -89.3572) (14.2622, -89.3488) (14.2241, -89.346) (14.1718, -89.3499) knots 0 0 0 0 1 1 1 1
  spline S1600 degree 3 poles (14.1718, -89.3499) (14.1195, -89.3538) (14.0728, -89.362) (14.0663, -89.3704) knots 0 0 0 0 1 1 1 1
  spline S1601 degree 3 poles (14.0663, -89.3704) (14.0598, -89.3787) (14.0978, -89.3816) (14.1501, -89.3777) knots 0 0 0 0 1 1 1 1
  spline S1602 degree 3 poles (11.5915, -92.6927) (11.615, -92.6797) (11.6318, -92.6525) (11.63, -92.6377) knots 0 0 0 0 1 1 1 1
  spline S1603 degree 3 poles (11.63, -92.6377) (11.6303, -92.62) (11.609, -92.6302) (11.5878, -92.6629) knots 0 0 0 0 1 1 1 1
  spline S1604 degree 3 poles (11.5878, -92.6629) (11.564, -92.6935) (11.5658, -92.7084) (11.5915, -92.6927) knots 0 0 0 0 1 1 1 1
  spline S1605 degree 3 poles (11.787, -92.4425) (11.8105, -92.4295) (11.8273, -92.4023) (11.8255, -92.3875) knots 0 0 0 0 1 1 1 1
  spline S1606 degree 3 poles (11.8255, -92.3875) (11.8258, -92.3698) (11.8044, -92.38) (11.7833, -92.4128) knots 0 0 0 0 1 1 1 1
  spline S1607 degree 3 poles (11.7833, -92.4128) (11.7594, -92.4433) (11.7613, -92.4582) (11.787, -92.4425) knots 0 0 0 0 1 1 1 1
  spline S1608 degree 3 poles (13.7136, -90.1827) (13.8903, -90.1686) (13.8903, -90.1686) (13.9102, -90.2692) knots 0 0 0 0 1 1 1 1
  line L118 (13.9102, -90.2692) -> (13.9329, -90.372)
  line L119 (13.9329, -90.372) -> (13.9306, -90.2717)
  spline S1609 degree 3 poles (13.9306, -90.2717) (13.9261, -90.2145) (13.9426, -90.1647) (13.9668, -90.1567) knots 0 0 0 0 1 1 1 1
  spline S1610 degree 3 poles (13.9668, -90.1567) (14.0649, -90.117) (13.892, -90.1206) (13.7205, -90.1568) knots 0 0 0 0 1 1 1 1
  line L120 (13.7205, -90.1568) -> (13.5369, -90.1969)
  line L121 (13.5369, -90.1969) -> (13.7136, -90.1827)
  spline S1611 degree 3 poles (12.8065, -91.3095) (12.8227, -91.3804) (12.8277, -91.3798) (12.8263, -91.307) knots 0 0 0 0 1 1 1 1
  spline S1612 degree 3 poles (12.8263, -91.307) (12.8264, -91.2668) (12.8215, -91.2272) (12.8159, -91.2229) knots 0 0 0 0 1 1 1 1
  spline S1613 degree 3 poles (12.8159, -91.2229) (12.7937, -91.2055) (12.7902, -91.2386) (12.8065, -91.3095) knots 0 0 0 0 1 1 1 1
  spline S1614 degree 3 poles (10.5849, -94.1357) (10.5905, -94.1401) (10.6301, -94.1352) (10.6713, -94.1226) knots 0 0 0 0 1 1 1 1
  spline S1615 degree 3 poles (10.6713, -94.1226) (10.74, -94.1091) (10.7394, -94.1042) (10.6667, -94.1056) knots 0 0 0 0 1 1 1 1
  spline S1616 degree 3 poles (10.6667, -94.1056) (10.594, -94.107) (10.5627, -94.1183) (10.5849, -94.1357) knots 0 0 0 0 1 1 1 1
  spline S1617 degree 3 poles (6.4654, -99.5574) (6.4594, -99.611) (6.4672, -99.6125) (6.4997, -99.5708) knots 0 0 0 0 1 1 1 1
  spline S1618 degree 3 poles (6.4997, -99.5708) (6.5193, -99.5458) (6.5228, -99.5127) (6.5089, -99.5018) knots 0 0 0 0 1 1 1 1
  spline S1619 degree 3 poles (6.5089, -99.5018) (6.4755, -99.4758) (6.4733, -99.4786) (6.4654, -99.5574) knots 0 0 0 0 1 1 1 1
  spline S1620 degree 3 poles (12.8026, -91.5035) (12.8115, -91.5552) (12.8257, -91.5886) (12.8365, -91.5747) knots 0 0 0 0 1 1 1 1
  spline S1621 degree 3 poles (12.8365, -91.5747) (12.8452, -91.5636) (12.8609, -91.5893) (12.8707, -91.6283) knots 0 0 0 0 1 1 1 1
  spline S1622 degree 3 poles (12.8707, -91.6283) (12.887, -91.6992) (12.8919, -91.6986) (12.8905, -91.6259) knots 0 0 0 0 1 1 1 1
  spline S1623 degree 3 poles (12.8905, -91.6259) (12.8879, -91.5835) (12.8786, -91.5494) (12.8638, -91.5512) knots 0 0 0 0 1 1 1 1
  spline S1624 degree 3 poles (12.8638, -91.5512) (12.8489, -91.5531) (12.8292, -91.5153) (12.8231, -91.4658) knots 0 0 0 0 1 1 1 1
  spline S1625 degree 3 poles (12.8231, -91.4658) (12.8149, -91.419) (12.8035, -91.3877) (12.797, -91.3961) knots 0 0 0 0 1 1 1 1
  spline S1626 degree 3 poles (12.797, -91.3961) (12.7905, -91.4044) (12.7938, -91.4518) (12.8026, -91.5035) knots 0 0 0 0 1 1 1 1
  spline S1627 degree 3 poles (15.7751, -87.6702) (15.789, -87.6811) (15.8332, -87.6932) (15.8663, -87.6967) knots 0 0 0 0 1 1 1 1
  spline S1628 degree 3 poles (15.8663, -87.6967) (15.8994, -87.7002) (15.9159, -87.6906) (15.902, -87.6798) knots 0 0 0 0 1 1 1 1
  spline S1629 degree 3 poles (15.902, -87.6798) (15.8853, -87.6667) (15.8438, -87.6567) (15.8107, -87.6533) knots 0 0 0 0 1 1 1 1
  spline S1630 degree 3 poles (15.8107, -87.6533) (15.7776, -87.6498) (15.7584, -87.6572) (15.7751, -87.6702) knots 0 0 0 0 1 1 1 1
  spline S1631 degree 3 poles (8.9114, -96.6559) (8.9318, -96.6584) (8.9566, -96.6554) (8.9631, -96.647) knots 0 0 0 0 1 1 1 1
  spline S1632 degree 3 poles (8.9631, -96.647) (8.9675, -96.6415) (8.9579, -96.6251) (8.944, -96.6142) knots 0 0 0 0 1 1 1 1
  spline S1633 degree 3 poles (8.944, -96.6142) (8.9273, -96.6012) (8.9053, -96.6064) (8.8923, -96.6231) knots 0 0 0 0 1 1 1 1
  spline S1634 degree 3 poles (8.8923, -96.6231) (8.8815, -96.637) (8.8882, -96.6512) (8.9114, -96.6559) knots 0 0 0 0 1 1 1 1
  spline S1635 degree 3 poles (10.975, -94.0375) (10.9806, -94.0419) (11.0202, -94.037) (11.0614, -94.0244) knots 0 0 0 0 1 1 1 1
  spline S1636 degree 3 poles (11.0614, -94.0244) (11.1301, -94.011) (11.1295, -94.006) (11.0568, -94.0074) knots 0 0 0 0 1 1 1 1
  spline S1637 degree 3 poles (11.0568, -94.0074) (10.984, -94.0088) (10.9528, -94.0202) (10.975, -94.0375) knots 0 0 0 0 1 1 1 1
  spline S1638 degree 3 poles (14.0652, -90.1396) (14.0708, -90.1439) (14.1104, -90.139) (14.1516, -90.1265) knots 0 0 0 0 1 1 1 1
  spline S1639 degree 3 poles (14.1516, -90.1265) (14.2203, -90.113) (14.2197, -90.108) (14.147, -90.1094) knots 0 0 0 0 1 1 1 1
  spline S1640 degree 3 poles (14.147, -90.1094) (14.0742, -90.1108) (14.043, -90.1222) (14.0652, -90.1396) knots 0 0 0 0 1 1 1 1
  spline S1641 degree 3 poles (15.9903, -87.7443) (16.0209, -87.7682) (16.0357, -87.7664) (16.02, -87.7407) knots 0 0 0 0 1 1 1 1
  spline S1642 degree 3 poles (16.02, -87.7407) (16.0071, -87.7171) (15.9799, -87.7004) (15.965, -87.7022) knots 0 0 0 0 1 1 1 1
  spline S1643 degree 3 poles (15.965, -87.7022) (15.9474, -87.7018) (15.9576, -87.7232) (15.9903, -87.7443) knots 0 0 0 0 1 1 1 1
  spline S1644 degree 3 poles (15.6228, -88.4152) (15.6172, -88.4511) (15.5923, -88.4944) (15.566, -88.5052) knots 0 0 0 0 1 1 1 1
  spline S1645 degree 3 poles (15.566, -88.5052) (15.5418, -88.5131) (15.565, -88.5178) (15.6167, -88.509) knots 0 0 0 0 1 1 1 1
  spline S1646 degree 3 poles (15.6167, -88.509) (15.7086, -88.5002) (15.713, -88.4946) (15.7027, -88.4105) knots 0 0 0 0 1 1 1 1
  spline S1647 degree 3 poles (15.7027, -88.4105) (15.6856, -88.2718) (15.6405, -88.2723) (15.6228, -88.4152) knots 0 0 0 0 1 1 1 1
  spline S1648 degree 3 poles (15.7225, -88.2648) (15.7411, -88.2524) (15.7671, -88.2191) (15.7768, -88.1953) knots 0 0 0 0 1 1 1 1
  spline S1649 degree 3 poles (15.7768, -88.1953) (15.7815, -88.1721) (15.765, -88.1816) (15.7346, -88.2206) knots 0 0 0 0 1 1 1 1
  spline S1650 degree 3 poles (15.7346, -88.2206) (15.7042, -88.2595) (15.6989, -88.2777) (15.7225, -88.2648) knots 0 0 0 0 1 1 1 1
  spline S1651 degree 3 poles (15.082, -89.2507) (15.1005, -89.2786) (15.111, -89.2823) (15.1151, -89.2542) knots 0 0 0 0 1 1 1 1
  spline S1652 degree 3 poles (15.1151, -89.2542) (15.1198, -89.231) (15.1988, -89.1987) (15.2922, -89.1822) knots 0 0 0 0 1 1 1 1
  spline S1653 degree 3 poles (15.2922, -89.1822) (15.4671, -89.1531) (15.4671, -89.1531) (15.2607, -89.1709) knots 0 0 0 0 1 1 1 1
  spline S1654 degree 3 poles (15.2607, -89.1709) (15.1512, -89.1794) (15.0571, -89.1909) (15.0549, -89.1937) knots 0 0 0 0 1 1 1 1
  spline S1655 degree 3 poles (15.0549, -89.1937) (15.0527, -89.1965) (15.0635, -89.2228) (15.082, -89.2507) knots 0 0 0 0 1 1 1 1
  spline S1656 degree 3 poles (5.5303, -101.6024) (5.5442, -101.6133) (5.607, -101.6131) (5.6735, -101.6024) knots 0 0 0 0 1 1 1 1
  line L122 (5.6735, -101.6024) -> (5.7945, -101.5851)
  line L123 (5.7945, -101.5851) -> (5.6708, -101.56)
  spline S1657 degree 3 poles (5.6708, -101.56) (5.557, -101.5338) (5.4774, -101.5612) (5.5303, -101.6024) knots 0 0 0 0 1 1 1 1
  spline S1658 degree 3 poles (11.8061, -93.6214) (11.8296, -93.6084) (11.8464, -93.5812) (11.8445, -93.5664) knots 0 0 0 0 1 1 1 1
  spline S1659 degree 3 poles (11.8445, -93.5664) (11.8449, -93.5487) (11.8235, -93.5589) (11.8024, -93.5916) knots 0 0 0 0 1 1 1 1
  spline S1660 degree 3 poles (11.8024, -93.5916) (11.7785, -93.6222) (11.7803, -93.6371) (11.8061, -93.6214) knots 0 0 0 0 1 1 1 1
  spline S1661 degree 3 poles (15.8259, -88.6366) (15.8871, -88.6844) (15.9137, -88.6962) (15.8819, -88.6624) knots 0 0 0 0 1 1 1 1
  spline S1662 degree 3 poles (15.8819, -88.6624) (15.8529, -88.6308) (15.8028, -88.5917) (15.7707, -88.5755) knots 0 0 0 0 1 1 1 1
  spline S1663 degree 3 poles (15.7707, -88.5755) (15.7391, -88.5643) (15.7626, -88.5916) (15.8259, -88.6366) knots 0 0 0 0 1 1 1 1
  spline S1664 degree 3 poles (5.6581, -101.7023) (5.6637, -101.7067) (5.7033, -101.7018) (5.7445, -101.6892) knots 0 0 0 0 1 1 1 1
  spline S1665 degree 3 poles (5.7445, -101.6892) (5.8132, -101.6758) (5.8126, -101.6708) (5.7399, -101.6722) knots 0 0 0 0 1 1 1 1
  spline S1666 degree 3 poles (5.7399, -101.6722) (5.6672, -101.6736) (5.6359, -101.685) (5.6581, -101.7023) knots 0 0 0 0 1 1 1 1
  spline S1667 degree 3 poles (5.9269, -101.599) (5.9464, -101.6142) (6.0801, -101.5978) (6.0953, -101.5783) knots 0 0 0 0 1 1 1 1
  spline S1668 degree 3 poles (6.0953, -101.5783) (6.104, -101.5672) (6.0724, -101.556) (6.0267, -101.5515) knots 0 0 0 0 1 1 1 1
  spline S1669 degree 3 poles (6.0267, -101.5515) (5.9478, -101.5436) (5.8908, -101.5707) (5.9269, -101.599) knots 0 0 0 0 1 1 1 1
  spline S1670 degree 3 poles (14.0345, -91.3019) (14.0549, -91.3045) (14.0797, -91.3014) (14.0862, -91.2931) knots 0 0 0 0 1 1 1 1
  spline S1671 degree 3 poles (14.0862, -91.2931) (14.0906, -91.2875) (14.081, -91.2711) (14.0671, -91.2602) knots 0 0 0 0 1 1 1 1
  spline S1672 degree 3 poles (14.0671, -91.2602) (14.0504, -91.2472) (14.0284, -91.2524) (14.0154, -91.2691) knots 0 0 0 0 1 1 1 1
  spline S1673 degree 3 poles (14.0154, -91.2691) (14.0045, -91.283) (14.0113, -91.2973) (14.0345, -91.3019) knots 0 0 0 0 1 1 1 1
  spline S1674 degree 3 poles (16.0105, -88.8301) (16.0494, -88.8605) (16.0677, -88.8658) (16.0547, -88.8422) knots 0 0 0 0 1 1 1 1
  spline S1675 degree 3 poles (16.0547, -88.8422) (16.0424, -88.8236) (16.009, -88.7976) (15.9852, -88.7879) knots 0 0 0 0 1 1 1 1
  spline S1676 degree 3 poles (15.9852, -88.7879) (15.9621, -88.7832) (15.9716, -88.7997) (16.0105, -88.8301) knots 0 0 0 0 1 1 1 1
  spline S1677 degree 3 poles (15.0556, -90.018) (15.0611, -90.0223) (15.1008, -90.0174) (15.1419, -90.0049) knots 0 0 0 0 1 1 1 1
  spline S1678 degree 3 poles (15.1419, -90.0049) (15.2106, -89.9914) (15.21, -89.9864) (15.1373, -89.9878) knots 0 0 0 0 1 1 1 1
  spline S1679 degree 3 poles (15.1373, -89.9878) (15.0646, -89.9892) (15.0333, -90.0006) (15.0556, -90.018) knots 0 0 0 0 1 1 1 1
  spline S1680 degree 3 poles (7.7772, -99.5974) (7.7911, -99.6083) (7.8159, -99.6052) (7.8289, -99.5886) knots 0 0 0 0 1 1 1 1
  spline S1681 degree 3 poles (7.8289, -99.5886) (7.8398, -99.5747) (7.8302, -99.5582) (7.8098, -99.5557) knots 0 0 0 0 1 1 1 1
  spline S1682 degree 3 poles (7.8098, -99.5557) (7.7866, -99.551) (7.7646, -99.5562) (7.7581, -99.5646) knots 0 0 0 0 1 1 1 1
  spline S1683 degree 3 poles (7.7581, -99.5646) (7.7538, -99.5701) (7.7605, -99.5844) (7.7772, -99.5974) knots 0 0 0 0 1 1 1 1
  spline S1684 degree 3 poles (6.263, -101.5929) (6.2769, -101.6038) (6.3016, -101.6007) (6.3146, -101.584) knots 0 0 0 0 1 1 1 1
  spline S1685 degree 3 poles (6.3146, -101.584) (6.3255, -101.5701) (6.3159, -101.5537) (6.2955, -101.5512) knots 0 0 0 0 1 1 1 1
  spline S1686 degree 3 poles (6.2955, -101.5512) (6.2723, -101.5465) (6.2504, -101.5517) (6.2438, -101.5601) knots 0 0 0 0 1 1 1 1
  spline S1687 degree 3 poles (6.2438, -101.5601) (6.2395, -101.5656) (6.2463, -101.5799) (6.263, -101.5929) knots 0 0 0 0 1 1 1 1
  spline S1688 degree 3 poles (15.336, -89.9685) (15.3694, -89.9945) (15.4496, -89.9721) (15.4453, -89.9374) knots 0 0 0 0 1 1 1 1
  spline S1689 degree 3 poles (15.4453, -89.9374) (15.4441, -89.9275) (15.4132, -89.9213) (15.3741, -89.9311) knots 0 0 0 0 1 1 1 1
  spline S1690 degree 3 poles (15.3741, -89.9311) (15.3324, -89.9387) (15.3193, -89.9554) (15.336, -89.9685) knots 0 0 0 0 1 1 1 1
  spline S1691 degree 3 poles (16.1256, -89.1125) (16.1518, -89.1822) (16.1546, -89.1843) (16.151, -89.1144) knots 0 0 0 0 1 1 1 1
  spline S1692 degree 3 poles (16.151, -89.1144) (16.1533, -89.0714) (16.1629, -89.0476) (16.1796, -89.0606) knots 0 0 0 0 1 1 1 1
  spline S1693 degree 3 poles (16.1796, -89.0606) (16.2129, -89.0867) (16.2198, -89.204) (16.1851, -89.2082) knots 0 0 0 0 1 1 1 1
  spline S1694 degree 3 poles (16.1851, -89.2082) (16.1703, -89.2101) (16.1696, -89.2453) (16.1772, -89.2871) knots 0 0 0 0 1 1 1 1
  spline S1695 degree 3 poles (16.1772, -89.2871) (16.1963, -89.3602) (16.1963, -89.3602) (16.1964, -89.2797) knots 0 0 0 0 1 1 1 1
  spline S1696 degree 3 poles (16.1964, -89.2797) (16.1967, -89.1591) (16.2272, -89.2232) (16.3116, -89.5219) knots 0 0 0 0 1 1 1 1
  spline S1697 degree 3 poles (16.3116, -89.5219) (16.3518, -89.6653) (16.3698, -89.7913) (16.3463, -89.8042) knots 0 0 0 0 1 1 1 1
  spline S1698 degree 3 poles (16.3463, -89.8042) (16.3233, -89.8221) (16.3301, -89.8363) (16.3666, -89.8469) knots 0 0 0 0 1 1 1 1
  spline S1699 degree 3 poles (16.3666, -89.8469) (16.4136, -89.8613) (16.4126, -89.874) (16.3705, -89.8992) knots 0 0 0 0 1 1 1 1
  spline S1700 degree 3 poles (16.3705, -89.8992) (16.3398, -89.9156) (16.3296, -89.9344) (16.35, -89.9369) knots 0 0 0 0 1 1 1 1
  spline S1701 degree 3 poles (16.35, -89.9369) (16.4057, -89.9402) (16.4011, -90.9259) (16.3456, -90.9453) knots 0 0 0 0 1 1 1 1
  spline S1702 degree 3 poles (16.3456, -90.9453) (16.3215, -90.9533) (16.3199, -90.961) (16.3431, -90.9657) knots 0 0 0 0 1 1 1 1
  spline S1703 degree 3 poles (16.3431, -90.9657) (16.3685, -90.9676) (16.3848, -91.1415) (16.3878, -91.3498) knots 0 0 0 0 1 1 1 1
  spline S1704 degree 3 poles (16.3878, -91.3498) (16.3882, -91.7217) (16.3781, -91.8033) (16.3474, -91.7166) knots 0 0 0 0 1 1 1 1
  spline S1705 degree 3 poles (16.3474, -91.7166) (16.3212, -91.647) (16.3017, -91.8152) (16.3231, -91.9081) knots 0 0 0 0 1 1 1 1
  spline S1706 degree 3 poles (16.3231, -91.9081) (16.3415, -91.9762) (16.3437, -91.9734) (16.3399, -91.8809) knots 0 0 0 0 1 1 1 1
  spline S1707 degree 3 poles (16.3399, -91.8809) (16.3354, -91.8237) (16.3469, -91.7745) (16.3618, -91.7727) knots 0 0 0 0 1 1 1 1
  spline S1708 degree 3 poles (16.3618, -91.7727) (16.3745, -91.7736) (16.3891, -91.8523) (16.3908, -91.9476) knots 0 0 0 0 1 1 1 1
  spline S1709 degree 3 poles (16.3908, -91.9476) (16.3907, -92.131) (16.3732, -92.1935) (16.3437, -92.1167) knots 0 0 0 0 1 1 1 1
  spline S1710 degree 3 poles (16.3437, -92.1167) (16.3329, -92.0904) (16.328, -92.091) (16.3217, -92.1219) knots 0 0 0 0 1 1 1 1
  spline S1711 degree 3 poles (16.3217, -92.1219) (16.3198, -92.1473) (16.3328, -92.1708) (16.3532, -92.1733) knots 0 0 0 0 1 1 1 1
  spline S1712 degree 3 poles (16.3532, -92.1733) (16.4067, -92.1793) (16.4002, -92.7607) (16.3469, -92.7773) knots 0 0 0 0 1 1 1 1
  spline S1713 degree 3 poles (16.3469, -92.7773) (16.3206, -92.7881) (16.319, -92.7958) (16.3422, -92.8005) knots 0 0 0 0 1 1 1 1
  spline S1714 degree 3 poles (16.3422, -92.8005) (16.4056, -92.8053) (16.4002, -94.7261) (16.3348, -94.7869) knots 0 0 0 0 1 1 1 1
  spline S1715 degree 3 poles (16.3348, -94.7869) (16.3016, -94.8236) (16.3012, -94.8413) (16.3356, -94.8546) knots 0 0 0 0 1 1 1 1
  spline S1716 degree 3 poles (16.3356, -94.8546) (16.3875, -94.8684) (16.4139, -94.9606) (16.3792, -95.0051) knots 0 0 0 0 1 1 1 1
  spline S1717 degree 3 poles (16.3792, -95.0051) (16.3683, -95.019) (16.3504, -94.9961) (16.3378, -94.9549) knots 0 0 0 0 1 1 1 1
  spline S1718 degree 3 poles (16.3378, -94.9549) (16.3244, -94.8862) (16.3194, -94.8868) (16.3208, -94.9595) knots 0 0 0 0 1 1 1 1
  spline S1719 degree 3 poles (16.3208, -94.9595) (16.3235, -95.0019) (16.3327, -95.0359) (16.3475, -95.0341) knots 0 0 0 0 1 1 1 1
  spline S1720 degree 3 poles (16.3475, -95.0341) (16.3822, -95.0299) (16.41, -95.1948) (16.3818, -95.231) knots 0 0 0 0 1 1 1 1
  spline S1721 degree 3 poles (16.3818, -95.231) (16.3687, -95.2477) (16.3496, -95.2148) (16.3374, -95.156) knots 0 0 0 0 1 1 1 1
  line L124 (16.3374, -95.156) -> (16.3175, -95.0554)
  line L125 (16.3175, -95.0554) -> (16.3204, -95.1606)
  spline S1722 degree 3 poles (16.3204, -95.1606) (16.3249, -95.2179) (16.3353, -95.2618) (16.3501, -95.26) knots 0 0 0 0 1 1 1 1
  spline S1723 degree 3 poles (16.3501, -95.26) (16.3826, -95.2585) (16.4065, -95.3712) (16.3805, -95.4045) knots 0 0 0 0 1 1 1 1
  spline S1724 degree 3 poles (16.3805, -95.4045) (16.3696, -95.4184) (16.3508, -95.4082) (16.34, -95.3819) knots 0 0 0 0 1 1 1 1
  spline S1725 degree 3 poles (16.34, -95.3819) (16.3292, -95.3555) (16.3215, -95.354) (16.3245, -95.3787) knots 0 0 0 0 1 1 1 1
  spline S1726 degree 3 poles (16.3245, -95.3787) (16.3276, -95.4035) (16.3411, -95.432) (16.3578, -95.445) knots 0 0 0 0 1 1 1 1
  spline S1727 degree 3 poles (16.3578, -95.445) (16.3995, -95.4776) (16.3987, -97.8452) (16.3594, -97.8324) knots 0 0 0 0 1 1 1 1
  spline S1728 degree 3 poles (16.3594, -97.8324) (16.3229, -97.8218) (16.2999, -98.1664) (16.3287, -98.2785) knots 0 0 0 0 1 1 1 1
  spline S1729 degree 3 poles (16.3287, -98.2785) (16.3379, -98.3126) (16.341, -98.2971) (16.3415, -98.2393) knots 0 0 0 0 1 1 1 1
  spline S1730 degree 3 poles (16.3415, -98.2393) (16.337, -98.182) (16.3485, -98.1328) (16.3634, -98.131) knots 0 0 0 0 1 1 1 1
  spline S1731 degree 3 poles (16.3634, -98.131) (16.3909, -98.1301) (16.4025, -98.4705) (16.3765, -98.5039) knots 0 0 0 0 1 1 1 1
  spline S1732 degree 3 poles (16.3765, -98.5039) (16.3656, -98.5178) (16.3487, -98.4822) (16.3364, -98.4233) knots 0 0 0 0 1 1 1 1
  line L126 (16.3364, -98.4233) -> (16.3165, -98.3227)